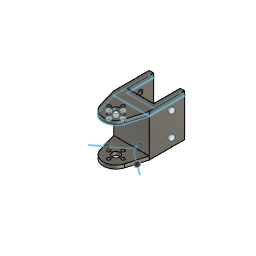
Servo arm connector (Autodesk Fusion 360 design; units mm, degrees)
Autodesk Fusion 360 part; units mm, degrees
sketch "sketch 1056" plane through (0, -11.0015, 8) normal (0, 0, 1) x (1, 0, 0)
  circle A0 centre (0, 8) radius 1.85
  circle A1 centre (0, 0) radius 4.4721
  circle A2 centre (-8, 0) radius 1.85
  circle A3 centre (8, 0) radius 1.85
  circle A4 centre (0, -8) radius 1.85
  line L0 (20, 17.4929) -> (-20, 17.4929)
  line L1 (-20, 17.4929) -> (-13.7579, -3.9964)
  arc A5 (-13.7579, -3.9964) -> (13.7579, -3.9964) centre (0, 0) ccw
  line L2 (20, 17.4929) -> (13.7579, -3.9964)
extrude "Extrude1" add sketch "sketch 1056" along normal blind 4 from surface at 0.5
sketch "sketch 1094" plane through (0, -11.0015, 8) normal (0, 0, 1) x (1, 0, 0)
  line L0 (-15, 27.4929) -> (15, 27.4929)
  line L1 (-15, 27.4929) -> (-15, 57.4929)
  line L2 (-15, 57.4929) -> (-20, 57.4929)
  line L3 (-20, 57.4929) -> (-20, 27.4929)
  line L4 (-20, 17.4929) -> (-20, 27.4929)
  line L5 (20, 17.4929) -> (-20, 17.4929)
  line L6 (20, 27.4929) -> (20, 17.4929)
  line L7 (20, 57.4929) -> (20, 27.4929)
  line L8 (15, 57.4929) -> (20, 57.4929)
  line L9 (15, 27.4929) -> (15, 57.4929)
extrude "Extrude2" add sketch "sketch 1094" along normal up to surface (4.5 mm away) and the other way up to surface (19.3 mm away)
mirror "Mirror1" about plane through (0, -26.35, -11.3) normal (0, 0, 1) of bodies 1 merged
sketch "sketch 1015" plane through (0, 10.5816, -35.1) normal (0, 0, -1) x (1, 0, 0)
  spline S0 degree 5 poles (0, -5.9097) (0, -5.175) (-0.0391, -3.7793) (-0.2151, -1.9064) (-0.6812, 0.1789) (-1.6353, 2.26) (-2.9441, 4.0116) (-4.59, 5.6249) (-6.5467, 7.2429) (-8.7784, 8.9432) (-11.252, 10.7641) (-13.4033, 12.3269) (-15.1068, 13.5582) (-16.2817, 14.405) (-16.8789, 14.8349) knots 0 0 0 0 0 0 0.1 0.2 0.3 0.4 0.5 0.6 0.7 0.8 0.9 1 1 1 1 1 1
  line L0 (-16.8789, 14.8349) -> (-28.8496, 23.4506)
  spline S1 degree 5 poles (0, -5.9097) (0, -5.175) (0.0391, -3.7793) (0.2151, -1.9064) (0.6812, 0.1789) (1.6353, 2.26) (2.9441, 4.0116) (4.59, 5.6249) (6.5467, 7.2429) (8.7784, 8.9432) (11.252, 10.7641) (13.4033, 12.3269) (15.1068, 13.5582) (16.2817, 14.405) (16.8789, 14.8349) knots 0 0 0 0 0 0 0.1 0.2 0.3 0.4 0.5 0.6 0.7 0.8 0.9 1 1 1 1 1 1
  line L1 (16.8789, 14.8349) -> (28.8496, 23.4506)
pipe "Pipe1" cut square section size 3 path "sketch 1015" along S0 L0
sketch "sketch 1040" plane through (20, 26.4913, -10.8) normal (1, 0, 0) x (0, 1, 0)
  circle A0 centre (5, -14.8) radius 2.65
  circle A1 centre (5, 11.8) radius 2.65
extrude "Extrude3" cut sketch "sketch 1040" against normal up to surface (5 mm away)
mirror "Mirror2" about plane through (0, 31.4929, -11.8) normal (1, 0, 0) of "Extrude3"
pipe "Pipe3" cut square section size 3 path "sketch 1015" along S1 L1
